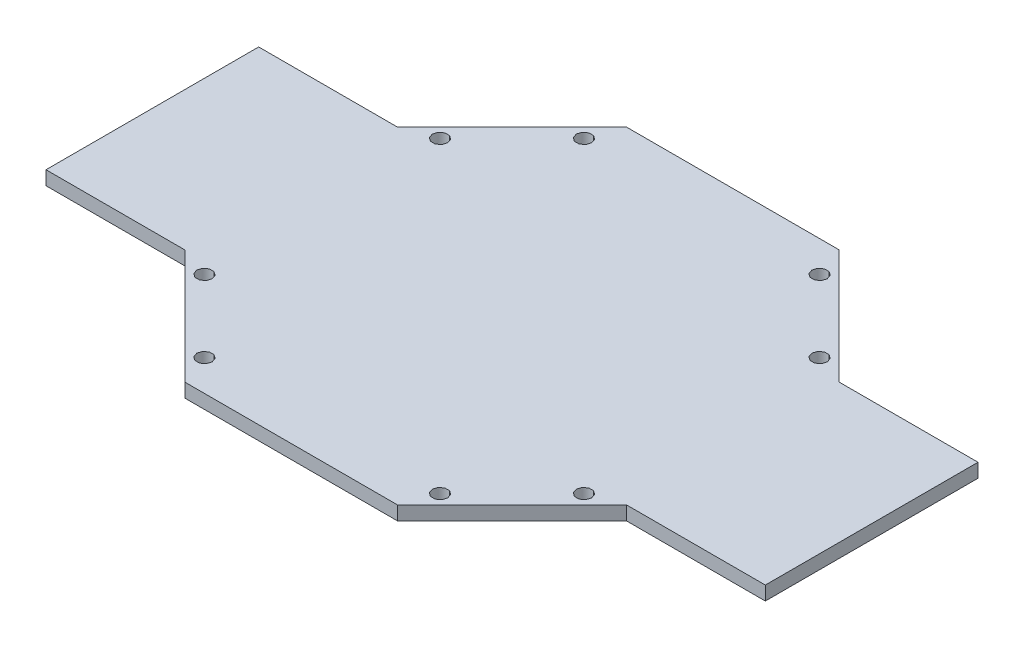
# Autodesk Inventor part: 下板
Saved by Autodesk Inventor 2025.2 (Build 292293000, 293)
## iProperties
Created: 2026-04-18
Part Number: 下板
Material: 常规
Document SubType Name: Modeling
Designer: BO‘S_SLAVE
Density: 1 g/cm^3
Appearance: 默认
Author: BO‘S_SLAVE
Autodesk Inventor part; units mm, degrees
ref_plane "YZ Plane" through (0, 0, 0) normal (1, 0, 0) x (0, 1, 0)
ref_plane "XZ Plane" through (0, 0, 0) normal (0, 1, 0) x (-1, 0, 0)
ref_plane "XY Plane" through (0, 0, 0) normal (0, 0, 1) x (1, 0, 0)
sketch "草图1" plane through (0, 0, 0) normal (0, 1, 0) x (-1, 0, 0)
  line L0 (35.3553, 35.3553) -> (-35.3553, 35.3553)
  line L1 (-35.3553, 35.3553) -> (-35.3553, -35.3553)
  line L2 (-35.3553, -35.3553) -> (35.3553, -35.3553)
  line L3 (35.3553, -35.3553) -> (35.3553, 35.3553)
  line L4 (35.3553, 35.3553) -> (-35.3553, -35.3553)
  line L5 (35.3553, -35.3553) -> (-35.3553, 35.3553)
  line L6 (-22.981, 47.7297) -> (-47.7297, 22.981)
  line L7 (-47.7297, -22.981) -> (-22.981, -47.7297)
  line L8 (22.981, -47.7297) -> (47.7297, -22.981)
  line L9 (47.7297, 22.981) -> (22.981, 47.7297)
  line L10 (22.981, 47.7297) -> (-22.981, 47.7297)
  line L11 (47.7297, 22.981) -> (47.7297, -22.981)
  line L12 (22.981, -47.7297) -> (-22.981, -47.7297)
  line L13 (-47.7297, -22.981) -> (-47.7297, 22.981)
  circle A0 centre (41.0122, 25.4558) radius 1.65
  circle A1 centre (25.4558, 41.0122) radius 1.65
  circle A2 centre (-41.0122, 25.4558) radius 1.65
  circle A3 centre (-25.4558, 41.0122) radius 1.65
  circle A4 centre (-25.4558, -41.0122) radius 1.65
  circle A5 centre (-41.0122, -25.4558) radius 1.65
  circle A6 centre (41.0122, -25.4558) radius 1.65
  circle A7 centre (25.4558, -41.0122) radius 1.65
  line L14 (-47.7297, -22.981) -> (-77.7297, -22.981)
  line L15 (-77.7297, -22.981) -> (-77.7297, 22.981)
  line L16 (-47.7297, 22.6987) -> (-47.7297, -22.981)
  line L17 (-47.7297, 22.981) -> (-77.7297, 22.981)
  line L18 (47.7297, -22.981) -> (77.7297, -22.981)
  line L19 (77.7297, -22.981) -> (77.7297, 22.981)
  line L20 (77.7297, 22.981) -> (47.7297, 22.981)
  point P0 (0, 0)
  point P1 (0, 0)
  point P2 (0, 0)
  point P3 (-35.3553, -35.3553)
  point P4 (35.3553, -35.3553)
  point P5 (35.3553, 35.3553)
  point P6 (0, 0)
  dimension "d4" = 100
  dimension "d5" = 35
  dimension "d6" = 45
  dimension "d7" = 360
  dimension "d8" = 3.3
  dimension "d9" = 3
  dimension "d10" = 11
  dimension "d18" = 360
  dimension "d20" = 30
  dimension "d23" = 30
  constraints: 42 end point, 9 perpendicular, 8 centre point, 4 parallel, 3 horizontal, 3 midpoint, 2 coincident, 1 symmetric about line, 35 other
  measures "d4" distance of L2.end L1.start
  measures "d5" distance of L6.start L6.end
  measures "d6" angle of L6 L1
  measures "d8" diameter of A0
  measures "d9" distance from line of L9 A0.centre
  measures "d10" distance from line of L4 A0.centre
  measures "d20" distance between parallel lines of L16 L15
  measures "d23" distance between parallel lines of L19 L11
extrude "拉伸1" add sketch "草图1" along normal blind 3
